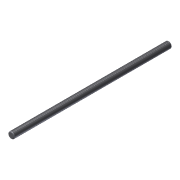
# Autodesk Inventor part: PS20011
Saved by Autodesk Inventor 2014 (Build 180170000, 170)
## iProperties
Category: NS
Created: 2011-09-26
Part Number: PS20011
Document SubType Name: Modeling
Designer: ERF
Density: 8 g/cm^3
Description: M8 Threaded Rod - Stainless Steel, 200mm
Material: Stainless Steel, Polished
Stock Number: S2TR-200
Vendor: NetBeef
Project: Shapeoko
Mass: 79.0173 g
Surface Area: 51.2708 cm^2
Volume: 10.0531 cm^3
Appearance: Steel
Catalog Web Link: http://www.mcmaster.com/#catalog/119/3147/=nu2cm7
Authority: PER ALEX BI @ NINGBO YINZHOU, 7-29-13 - INCLUDES SHIPPING
Title: Threaded Rod
Author: ERF
Subject: Motion
Comments: Fusion
Autodesk Inventor part; units mm, degrees
ref_plane "YZ Plane" through (0, 0, 0) normal (1, 0, 0) x (0, 1, 0)
ref_plane "XZ Plane" through (0, 0, 0) normal (0, 1, 0) x (-1, 0, 0)
ref_plane "XY Plane" through (0, 0, 0) normal (0, 0, 1) x (1, 0, 0)
sketch "Sketch1" plane through (0, 0, 0) normal (0, 0, 1) x (1, 0, 0)
  circle A0 centre (0, 0) radius 4
  dimension "d0" = 8
  constraints: 1 centre point
  measures "d0" diameter of A0
extrude "Extrusion1" add sketch "Sketch1" along normal blind 200
thread "Thread1" size "M8x1.25" class "6g" standard "ANSI Metric M Profile" full length
fillet "Fillet1" radius 1 2 edges at (-4, 0, 200) (-4, 0, 0)
body "Solid1"
